Autodesk Fusion 360 part; units mm, degrees
(part 2 of 2)
copy_body "CopyPasteBodies14" bodies 31 32 33 28 makes body 34 makes body 35 makes body 36 makes body 37
move_body "Move22" bodies 34 35 36 37 to x (-1, 0, 0) y (0, -1, 0) z (0, 0, 1) at (197.9996, 63.9485, 0)
hidden bodies 20 27 28 29 1 2 3 4 5 6 7 8 9 10 11 12 13 14 15 16 17 18 30
equation "tile_size = 200 mm"
equation "wall_tab_height = 14 mm"
equation "wall_width = 12.34 mm"
equation "wall_tab_radius = 2.0 mm"
equation "d6 = tile_size"
equation "wall_tab_angle = 70 deg"
equation "wall_height = 70 mm"
equation "wall_tab_base = 30 mm"
equation "d11 = wall_tab_angle"
equation "d12 = wall_tab_height"
equation "d13 = wall_tab_angle"
equation "d14 = wall_tab_base"
equation "d15 = wall_height"
equation "d18 = ( wall_height - wall_tab_base ) / 2"
equation "d22 = wall_height / 2 + wall_gap_extra"
equation "wall_notch_notch = 3.2 mm"
equation "d24 = wall_notch_notch"
equation "d25 = wall_notch_notch"
equation "d26 = wall_notch_notch / 2"
equation "d27 = wall_notch_notch / 2"
equation "d28 = wall_width"
equation "d30 = wall_tab_radius"
equation "d31 = wall_tab_radius"
equation "d34 = tile_size"
equation "d35 = wall_tab_height"
equation "d36 = wall_tab_angle"
equation "d37 = wall_tab_height"
equation "d38 = wall_tab_angle"
equation "d39 = wall_tab_base"
equation "d41 = wall_tab_base"
equation "d42 = ( wall_height - wall_tab_base ) / 2"
equation "d43 = ( wall_height - wall_tab_base ) / 2"
equation "d44 = wall_width + 2 * wall_notch_notch"
equation "d51 = wall_tab_radius"
equation "d52 = wall_tab_radius"
equation "d53 = wall_tab_radius"
equation "d54 = wall_tab_radius"
equation "d55 = ( tile_size - wall_width ) * 0.5"
equation "d56 = wall_height / 2"
equation "d57 = wall_notch_notch"
equation "d58 = wall_notch_notch"
equation "d59 = wall_notch_notch"
equation "d60 = wall_notch_notch"
equation "d61 = wall_height"
equation "d62 = wall_width"
equation "d64 = -tile_size / 2"
equation "d66 = -wall_width / 2"
equation "d67 = -wall_width / 2"
equation "d69 = -tile_size / 2"
equation "d70 = tile_size"
equation "d75 = tile_size"
equation "d76 = tile_size"
equation "d79 = tile_size"
equation "d84 = tile_size"
equation "d87 = tile_size"
equation "d90 = wall_notch_notch / 2"
equation "d91 = wall_notch_notch"
equation "d92 = wall_notch_notch / 2"
equation "d93 = wall_notch_notch"
equation "d94 = 20 mm - wall_width_gap / 2"
equation "d95 = wall_width_gap"
equation "d97 = wall_width_extrude"
equation "d109 = 5 mm + 1.57 mm"
equation "d113 = wall_tab_height"
equation "d114 = wall_tab_base"
equation "d116 = wall_tab_angle"
equation "d117 = wall_tab_angle"
equation "d122 = wall_tab_height"
equation "d123 = wall_tab_base"
equation "d124 = wall_tab_angle"
equation "d125 = wall_tab_angle"
equation "d126 = 25 mm - wall_tab_base / 2"
equation "d127 = wall_tab_radius"
equation "d128 = wall_tab_radius"
equation "d160 = wall_tab_radius"
equation "d161 = wall_tab_radius"
equation "d185 = wall_tab_height"
equation "d186 = wall_tab_base"
equation "d187 = wall_tab_angle"
equation "d188 = wall_tab_angle"
equation "d189 = 25 mm - wall_tab_base / 2"
equation "d190 = wall_tab_radius"
equation "d191 = wall_tab_radius"
equation "d195 = wall_width_extrude"
equation "wall_width_extrude = 12.30 mm"
equation "wall_width_gap = 12.4 mm"
equation "d199 = tile_size / 2"
equation "d200 = wall_width_gap"
equation "d201 = wall_tab_angle"
equation "d202 = wall_tab_angle"
equation "d203 = wall_tab_base"
equation "d204 = ( wall_height - wall_tab_base ) / 2"
equation "d205 = wall_tab_height"
equation "d206 = wall_tab_radius"
equation "d207 = wall_tab_radius"
equation "d208 = wall_tab_radius"
equation "d209 = wall_tab_radius"
equation "d210 = wall_tab_radius"
equation "d211 = wall_width_extrude"
equation "d213 = wall_tab_angle"
equation "d214 = wall_tab_height"
equation "d215 = wall_tab_angle"
equation "d216 = wall_tab_base"
equation "d217 = ( wall_height - wall_tab_base ) / 2"
equation "d218 = wall_tab_radius"
equation "d219 = wall_tab_radius"
equation "d220 = wall_tab_radius"
equation "d221 = wall_height"
equation "d223 = wall_tab_radius"
equation "d224 = wall_tab_radius"
equation "utab_sub_extrude = 6.12 mm"
equation "d228 = tab_screw_diam"
equation "tab_screw_diam = 5.8 mm"
equation "d230 = tab_screw_diam"
equation "bstrip_width = light_holder_tab_width * 4 + 2 mm"
equation "bstrip_height = 3.65 mm"
equation "d233 = bstrip_height"
equation "d234 = bstrip_width + bstrip_extra_for_tool"
equation "d237 = bstrip_width + bstrip_extra_for_tool"
equation "d238 = bstrip_height"
equation "bstrip_from_buttom = 9 mm"
equation "d241 = tile_size / 4"
equation "d242 = tile_size / 4"
equation "bstrip_extra_for_tool = 3.2 mm" comment "3.2/2"
equation "wire_notch_width = 5 mm"
equation "wire_notch_height = 2.2 mm"
equation "d246 = wire_notch_width"
equation "d247 = wire_notch_height"
equation "d248 = bstrip_from_buttom"
equation "d249 = bstrip_from_buttom"
equation "d250 = wire_notch_width"
equation "d251 = wire_notch_height"
equation "d252 = btn_holder_width"
equation "btn_holder_width = 14 mm"
equation "btn_holder_cutter_height = 20 mm"
equation "btn_holder_cut_depth = 1 mm"
equation "btn_holder_cut_height = 16 mm"
equation "d257 = wall_notch_notch / 2"
equation "d258 = wall_notch_notch / 2"
equation "d259 = btn_holder_cutter_height"
equation "d260 = btn_holder_cut_height"
equation "d261 = btn_holder_from_gap"
equation "btn_holder_from_gap = 7 mm"
equation "d263 = wall_notch_notch"
equation "d264 = btn_holder_width"
equation "d265 = wall_notch_notch"
equation "d266 = wall_notch_notch / 2"
equation "d267 = wall_notch_notch / 2"
equation "d268 = btn_holder_cutter_height"
equation "d269 = btn_holder_cut_height"
equation "d270 = btn_holder_from_gap"
equation "d271 = btn_holder_width"
equation "d272 = wall_notch_notch / 2"
equation "d273 = wall_notch_notch / 2"
equation "d274 = wall_notch_notch"
equation "d275 = btn_holder_cutter_height"
equation "d276 = btn_holder_cut_height"
equation "d277 = btn_holder_from_gap"
equation "d278 = wall_notch_notch / 2"
equation "d279 = wall_notch_notch / 2"
equation "d280 = wall_notch_notch"
equation "d281 = btn_holder_width"
equation "d282 = btn_holder_cutter_height"
equation "d283 = btn_holder_cut_height"
equation "d284 = btn_holder_from_gap"
equation "d289 = wall_height / 2"
equation "btn_holder_hole_diam = 3.4 mm"
equation "d292 = btn_holder_hole_diam"
equation "d293 = btn_holder_hole_diam"
equation "d294 = btn_holder_hole_diam"
equation "d295 = btn_holder_hole_diam"
equation "d296 = bstrip_width + bstrip_extra_for_tool"
equation "d297 = bstrip_height"
equation "d298 = wire_notch_width"
equation "d299 = wire_notch_height"
equation "d301 = bstrip_from_buttom"
equation "d302 = bstrip_width + bstrip_extra_for_tool"
equation "d303 = bstrip_height"
equation "d304 = wire_notch_height"
equation "d305 = wire_notch_width"
equation "d306 = bstrip_from_buttom"
equation "wall_gap_extra = 0.15 mm"
equation "d308 = tile_size - wall_width_gap - 0.38 mm"
equation "light_holder_width = 30 mm"
equation "light_holder_tab_len = 11 mm"
equation "d311 = light_holder_width"
equation "light_holder_tab_width = 6 mm"
equation "d315 = light_holder_tab_width"
equation "d316 = light_holder_tab_len"
equation "d317 = light_holder_tab_len"
equation "d318 = light_holder_tab_width"
equation "light_holder_extrude = 3.87 mm"
equation "d320 = light_holder_extrude"
equation "d322 = light_holder_tab_width"
equation "d323 = light_holder_tab_width"
equation "d326 = light_holder_tab_len"
equation "d327 = light_holder_tab_width"
equation "d328 = light_holder_tab_width"
equation "d331 = btn_bridge_thickness"
equation "d334 = btn_bridge_thickness"
equation "d335 = btn_bridge_thickness"
equation "d336 = btn_bridge_thickness"
equation "d337 = btn_bridge_thickness"
equation "d340 = btn_bridge_thickness"
equation "d348 = btn_holder_hole_diam_plastic"
equation "d352 = btn_holder_hole_diam_plastic"
equation "d353 = btn_extrude"
equation "d355 = wall_height / 2 + 1 mm"
equation "d362 = btn_bridge_thickness"
equation "d363 = btn_bridge_thickness"
equation "d364 = btn_bridge_thickness"
equation "d365 = btn_bridge_thickness"
equation "btn_extrude = 5.4 mm"
equation "btn_bridge_thickness = 1.5 mm"
equation "btn_holder_hole_diam_plastic = 4.10 mm"
equation "d381 = wall_width_extrude"
named bodies: "wall_up1", "wall_down1", "wall_up2", "wall_down2", "wall_down1 (1)", "wall_down3", "wall_down4", "wall_up3", "wall_up1 (1)", "wall_up4", "wall_tester", "simple_block", "test_hole", "test_tab_in", "test_tab_out", "test_tab_sq_in", "test_tab_sq_out", "test_tab_sq2", "test_tab_out2", "test_utab", "test_utab (1)", "wall_utab", "utab_cutter", "utab_cutter (1)", "btn_cutter1", "btn_cutter2", "btn_cutter3", "btn_cutter4", "light_holder", "button", "button_moved", "bore_test", "button (1)", "button copy1", "button (2)", "button copy2", "button (3)", "button copy3", "button (1) (1)", "button (2) (1)", "button (3) (1)", "button (4)", "button copy4", "button copy5", "button copy6", "button copy7"
